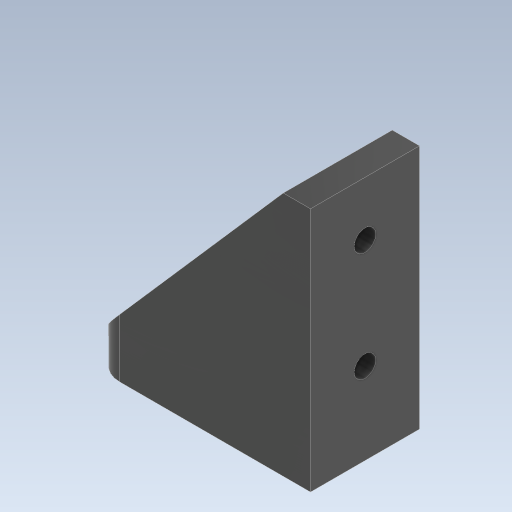
# Autodesk Inventor part: INDX_005_Cornerbracket
Saved by Autodesk Inventor 2024 (Build 280153000, 153)
## iProperties
Created: 2024-08-08
Part Number: INDX_005_Cornerbracket
Material: ABS Plastic
Document SubType Name: Modeling
Designer: Oscar
Density: 1.06 g/cm^3
Appearance: Dark Gray
Author: Oscar
Autodesk Inventor part; units mm, degrees
ref_plane "YZ Plane" through (0, 0, 0) normal (1, 0, 0) x (0, 1, 0)
ref_plane "XZ Plane" through (0, 0, 0) normal (0, 1, 0) x (-1, 0, 0)
ref_plane "XY Plane" through (0, 0, 0) normal (0, 0, 1) x (1, 0, 0)
sketch "Sketch1" plane through (0, 0, 0) normal (0, 1, 0) x (-1, 0, 0)
  line L0 (0, 0) -> (50.8, 0)
  line L1 (50.8, 0) -> (50.8, -25.4)
  line L2 (50.8, -25.4) -> (0, -25.4)
  line L3 (0, -25.4) -> (0, 0)
  circle A0 centre (19.05, -12.7) radius 3.2639
  circle A1 centre (44.45, -12.7) radius 3.2639
  point P0 (0, -12.7)
  dimension "d0" = 50.8
  dimension "d1" = 25.4
  dimension "d2" = 6.5278
  dimension "d3" = 25.4
  dimension "d4" = 19.05
  dimension "d5" = 12.7
  constraints: 8 end point, 2 centre point, 2 parallel, 1 equal radius, 1 horizontal, 1 horizontal alignment, 1 midpoint, 1 perpendicular
  measures "d0" distance of L1.end L2.end
  measures "d1" distance of L0.end L1.end
  measures "d2" diameter of A0
  measures "d3" distance of A0.centre A1.centre
  measures "d4" distance of point (0, -12.7) A0.centre
  measures "d5" distance from line of L0 A0.centre
extrude "Extrusion1" add sketch "Sketch1" along normal blind 6.35
sketch "Sketch2" plane through (0, 6.35, 0) normal (0, 1, 0) x (1, 0, 0)
  line L0 (0, 25.4) -> (-50.8, 25.4) projected
  line L1 (0, 0) -> (-6.35, 0)
  line L2 (-6.35, 0) -> (-6.35, 25.4)
  line L3 (-6.35, 25.4) -> (0, 25.4)
  line L4 (0, 25.4) -> (0, 0)
  dimension "d8" = 6.35
  constraints: 8 end point, 2 parallel, 1 horizontal, 1 perpendicular, 1 point on line
  measures "d8" distance of L2.end L3.end
extrude "Extrusion2" add sketch "Sketch2" along normal blind 50.8
sketch "Sketch3" plane through (-6.35, 6.35, -25.4) normal (-1, 0, 0) x (0, 0, 1)
  circle A0 centre (12.7, 12.7) radius 2.4892
  circle A1 centre (12.7, 38.1) radius 2.4892
  line L0 (0, 0) -> (25.4, 0) projected
  line L1 (25.4, 0) -> (25.4, 50.8) projected
  point P0 (25.4, -6.35)
  dimension "d11" = 4.9784
  dimension "d12" = 4.9784
  dimension "d13" = 25.4
  dimension "d14" = 12.7
  dimension "d15" = 12.7
  constraints: 2 centre point, 1 vertical alignment
  measures "d11" diameter of A0
  measures "d12" diameter of A1
  measures "d13" distance of A1.centre A0.centre
  measures "d14" distance from line of A0.centre L0
  measures "d15" distance from line of L1 A1.centre
extrude "Extrusion3" cut sketch "Sketch3" against normal through all
sketch "Sketch4" plane through (-50.8, 0, 0) normal (0, 0, 1) x (1, 0, 0)
  line L0 (0, 6.35) -> (44.45, 6.35) projected
  line L1 (0, 0) -> (50.8, 0) projected
  line L2 (50.8, 0) -> (50.8, 57.15) projected
  line L3 (44.45, 57.15) -> (50.8, 57.15) projected
  line L4 (44.45, 6.35) -> (44.45, 57.15) projected
  line L5 (0, 6.35) -> (44.45, 6.35) projected
  line L6 (0, 0) -> (0, 6.35) projected
  line L7 (0, 6.35) -> (44.45, 57.15)
  line L8 (50.8, 57.15) -> (50.8, 0)
  line L9 (0, 0) -> (0, 6.35)
  line L10 (50.8, 0) -> (0, 0)
  line L11 (44.45, 57.15) -> (50.8, 57.15)
  constraints: 10 end point, 2 parallel, 1 collinear, 1 perpendicular
extrude "Extrusion4" add sketch "Sketch4" against normal blind 3.175 contours L7 L4 L0
sketch "Sketch5" plane through (0, 0, -25.4) normal (0, 0, -1) x (-1, 0, 0)
  line L0 (0, 0) -> (50.8, 0) projected
  line L1 (50.8, 0) -> (50.8, 6.35) projected
  line L2 (6.35, 6.35) -> (50.8, 6.35) projected
  line L3 (6.35, 6.35) -> (6.35, 57.15) projected
  line L4 (0, 57.15) -> (6.35, 57.15) projected
  line L5 (0, 0) -> (0, 57.15) projected
  line L6 (50.8, 6.35) -> (50.8, 0)
  line L7 (0, 0) -> (50.8, 0)
  line L8 (50.8, 6.35) -> (6.35, 57.15)
  line L9 (0, 0) -> (0, 57.15) projected
  line L10 (6.35, 57.15) -> (0, 57.15)
  line L11 (0, 57.15) -> (0, 0)
  constraints: 10 end point, 1 collinear, 1 horizontal, 1 perpendicular, 1 vertical
extrude "Extrusion5" add sketch "Sketch5" against normal blind 3.175
fillet "Fillet1" radius 6.35 2 edges at (-50.8, 3.175, -25.4) (-50.8, 3.175, 0)
body "Solid1"
